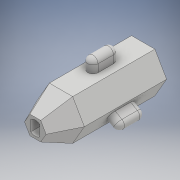
# Autodesk Inventor part: acopladorV5
Saved by Autodesk Inventor 2018.2 (Build 222227000, 227)
## iProperties
Created: 2018-01-25
Part Number: acopladorV5
Material: Genérico
Document SubType Name: Modeling
Designer: alber
Density: 1 g/cm^3
Appearance: Valor por defecto
Author: alber
Autodesk Inventor part; units mm, degrees
ref_plane "YZ Plane" through (0, 0, 0) normal (1, 0, 0) x (0, 1, 0)
ref_plane "XZ Plane" through (0, 0, 0) normal (0, 1, 0) x (-1, 0, 0)
ref_plane "XY Plane" through (0, 0, 0) normal (0, 0, 1) x (1, 0, 0)
sketch "Boceto11" plane through (0, 0, 0) normal (0, 1, 0) x (-1, 0, 0)
  line L0 (0, 0) -> (5.6, 0)
  line L1 (5.6, 0) -> (2.8, -4.8497)
  line L2 (2.8, -4.8497) -> (-2.8, -4.8497)
  line L3 (-2.8, -4.8497) -> (-5.6, 0)
  line L4 (-5.6, 0) -> (-2.8, 4.8497)
  line L5 (-2.8, 4.8497) -> (2.8, 4.8497)
  line L6 (2.8, 4.8497) -> (5.6, 0)
  line L7 (5.6, 0) -> (9.1, 0)
  line L8 (9.1, 0) -> (4.55, -7.8808)
  line L9 (4.55, -7.8808) -> (-4.55, -7.8808)
  line L10 (-4.55, -7.8808) -> (-9.1, 0)
  line L11 (-9.1, 0) -> (-4.55, 7.8808)
  line L12 (-4.55, 7.8808) -> (4.55, 7.8808)
  line L13 (4.55, 7.8808) -> (9.1, 0)
  dimension "d42" = 5.6
  dimension "d43" = 3.5
  constraints: 28 end point, 2 coincident, 1 horizontal, 1 point on line, 26 other
  measures "d42" distance of L0.start L0.end
  measures "d43" distance of L0.end L7.end
extrude "Extrusión10" add sketch "Boceto11" along normal blind 32
sketch "Boceto12" plane through (-8.8625, 0, -0.4114) normal (-0.8660254, 0, -0.5) x (-0.5, 0, 0.8660254)
  line L0 (0, 0) -> (0, 32)
  line L1 (0, 0) -> (0, 16)
  line L2 (-1.75, 32) -> (1.15, 32)
  line L3 (-9.3, 32) -> (-9.3, 0)
  line L4 (-4.65, 11) -> (-6.65, 11)
  line L5 (-6.65, 11) -> (-2.65, 11)
  line L6 (-2.65, 11) -> (-2.65, 21)
  line L7 (-2.65, 21) -> (-4.65, 21)
  line L8 (-4.65, 21) -> (-6.65, 21)
  line L9 (-6.65, 21) -> (-6.65, 11)
  point P0 (-4.65, 2)
  constraints: 20 end point, 3 perpendicular, 2 point on line, 1 horizontal
extrude "Extrusión11" add sketch "Boceto12" along normal blind 5
sketch "Boceto13" plane through (4.075, 0, 7.8808) normal (0, 0, 1) x (1, 0, 0)
  line L0 (0, 0) -> (0, 32)
  line L1 (0, 0) -> (0, 16)
  line L2 (-1.75, 32) -> (1.15, 32)
  line L3 (-9.3, 32) -> (-9.3, 0)
  line L4 (-4.65, 11) -> (-6.65, 11)
  line L5 (-6.65, 11) -> (-2.65, 11)
  line L6 (-2.65, 11) -> (-2.65, 21)
  line L7 (-2.65, 21) -> (-4.65, 21)
  line L8 (-4.65, 21) -> (-6.65, 21)
  line L9 (-6.65, 21) -> (-6.65, 11)
  point P0 (-4.65, 2)
  constraints: 20 end point, 3 perpendicular, 2 point on line, 1 horizontal
extrude "Extrusión12" add sketch "Boceto13" along normal blind 5
sketch "Boceto14" plane through (4.7875, 0, -7.4695) normal (0.8660254, 0, -0.5) x (-0.5, 0, -0.8660254)
  line L0 (0, 0) -> (0, 32)
  line L1 (0, 0) -> (0, 16)
  line L2 (-1.75, 32) -> (1.15, 32)
  line L3 (-9.3, 32) -> (-9.3, 0)
  line L4 (-4.65, 11) -> (-6.65, 11)
  line L5 (-6.65, 11) -> (-2.65, 11)
  line L6 (-2.65, 11) -> (-2.65, 21)
  line L7 (-2.65, 21) -> (-4.65, 21)
  line L8 (-4.65, 21) -> (-6.65, 21)
  line L9 (-6.65, 21) -> (-6.65, 11)
  point P0 (-4.65, 2)
  constraints: 20 end point, 3 perpendicular, 2 point on line, 1 horizontal
extrude "Extrusión13" add sketch "Boceto14" along normal blind 5
fillet "Empalme7" radius 2 6 edges at (12.4426, 16, -4.2104) (10.4426, 16, -7.6745) (1.425, 16, 12.8808) (-9.8676, 16, -8.6704) (-11.8676, 16, -5.2063) (-2.575, 16, 12.8808)
fillet "Empalme8" radius 2 18 edges at (1.425, 11, 9.3809) (-2.575, 11, 9.3809) (0.8392, 11, 12.2951) (-2.575, 21, 9.3809) (1.425, 21, 9.3809) (0.8392, 21, 12.2951) (9.4116, 21, -2.4604) (7.4116, 21, -5.9245) (11.6425, 21, -4.4248) (7.4116, 11, -5.9245) (9.4116, 11, -2.4604) (11.6425, 11, -4.4248) (-6.8366, 21, -6.9205) (-8.8366, 21, -3.4564) (-9.6532, 21, -7.8703) (-8.8366, 11, -3.4564) (-6.8366, 11, -6.9205) (-9.6532, 11, -7.8703)
sketch "Boceto16" plane through (0, 0, 0) normal (0, -1, 0) x (1, 0, 0)
  line L0 (4.55, 7.8808) -> (9.1, 0) projected
  line L1 (9.1, 0) -> (4.55, -7.8808)
  line L2 (4.55, -7.8808) -> (-4.55, -7.8808)
  line L3 (-4.55, -7.8808) -> (-9.1, 0)
  line L4 (-9.1, 0) -> (-4.55, 7.8808)
  line L5 (-4.55, 7.8808) -> (4.55, 7.8808)
  line L6 (4.55, 7.8808) -> (9.1, 0)
  point P0 (0, 0)
  point P1 (0, 0)
  constraints: 12 end point, 1 coincident, 13 other
extrude "Extrusión14" add sketch "Boceto16" along normal blind 10 draft -23
sketch "Boceto17" plane through (0, -10, 0) normal (0, -1, 0) x (1, 0, 0)
  line L0 (1.725, 0) -> (1.725, -2.1095)
  line L1 (1.725, 2.1095) -> (1.725, 0)
  line L2 (-1.725, 0) -> (-1.725, -2.1095)
  line L3 (-1.725, 0) -> (-1.725, 2.1095)
  arc A0 (1.725, 2.1095) -> (-1.725, 2.1095) centre (0, 0) ccw
  arc A1 (-1.725, -2.1095) -> (1.725, -2.1095) centre (0, 0) ccw
  constraints: 8 end point, 4 point on circle, 2 centre point, 2 equal length, 2 point on line, 1 coincident
extrude "Extrusión15" cut sketch "Boceto17" against normal blind 5
sketch "Boceto18" plane through (1.725, -10, -2.1095) normal (-1, 0, 0) x (0, 0, 1)
  point P0 (2.1095, 10)
